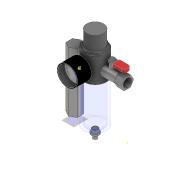
# Autodesk Inventor part: salida_estanque
Saved by Autodesk Inventor 2022 (Build 260153000, 153)
## iProperties
Created: 2022-11-16
Part Number: salida_estanque
Material: Generic
Document SubType Name: Modeling
Designer: ferna
Density: 1 g/cm^3
Appearance: Galvanized
Author: ferna
Autodesk Inventor part; units mm, degrees
ref_plane "YZ Plane" through (0, 0, 0) normal (1, 0, 0) x (0, 1, 0)
ref_plane "XZ Plane" through (0, 0, 0) normal (0, 1, 0) x (-1, 0, 0)
sketch "Sketch1" plane through (0, 0, 0) normal (0, 1, 0) x (-1, 0, 0)
  line L0 (-8, 4.6188) -> (0, 9.2376)
  line L1 (0, 9.2376) -> (8, 4.6188)
  line L2 (8, 4.6188) -> (8, -4.6188)
  line L3 (8, -4.6188) -> (0, -9.2376)
  line L4 (0, -9.2376) -> (-8, -4.6188)
  line L5 (-8, -4.6188) -> (-8, 4.6188)
  point P0 (0, 0)
  point P1 (0, 0)
  dimension "d0" = 8
  constraints: 12 end point, 1 coincident, 13 other
  measures "d0" distance from line of L5 point (0, 0)
extrude "Extrusion1" add sketch "Sketch1" along normal blind 85
sketch "Sketch2" plane through (0, 0, 0) normal (0, -1, 0) x (1, 0, 0)
  circle A0 centre (0, 0) radius 2.5
  dimension "d3" = 5
  constraints: 1 centre point, 1 coincident
  measures "d3" diameter of A0
extrude "Extrusion2" cut sketch "Sketch2" against normal blind 3
sketch "Sketch3" plane through (8, 0, 4.6188) normal (1, 0, 0) x (0, 0, -1)
  circle A0 centre (4.6188, 74.0681) radius 4.2105
  point P0 (4.6188, 0)
  dimension "d22" = 8.4209
  constraints: 1 centre point
  measures "d22" diameter of A0
extrude "Extrusion3" add sketch "Sketch3" along normal blind 5
sketch "Sketch4" plane through (0, 85, 0) normal (0, 1, 0) x (1, 0, 0)
  circle A0 centre (28.9651, 0) radius 15.9651
  point P0 (0, 0)
  constraints: 1 centre point
extrude "Extrusion4" add sketch "Sketch4" along normal blind 10 and the other way blind 25
sketch "Sketch6" plane through (0, 85, 0) normal (0, 1, 0) x (1, 0, 0)
  line L0 (8, 4.5892) -> (13, 4.5892)
  line L1 (13, 4.5892) -> (13, -4.9795)
  line L2 (13, -4.9795) -> (8, -4.9795)
  line L3 (8, -4.9795) -> (8, 4.5892)
  point P0 (0, 0)
  constraints: 8 end point, 2 parallel, 1 horizontal, 1 perpendicular
split body "Split1" sketch "Sketch6" result two bodies curves L2 L3 L0 L1 first body at (-5.0833, 28.3333, 5.7254) (13.7003, 77.7595, -2.4808)
sketch "Sketch7" plane through (28.9651, 95, 0) normal (0, 1, 0) x (1, 0, 0)
  circle A0 centre (0, 0) radius 17.3739
  point P0 (-28.9651, 0)
  constraints: 1 centre point
split body "Split2" sketch "Sketch7" result two bodies bodies 2 curves A0 first body at (44.2299, 71.6667, 2.4808)
sketch "Sketch8" plane through (13, 74.0681, 0) normal (1, 0, 0) x (0, 0, -1)
  circle A0 centre (0, 0) radius 4.2105 projected
  point P0 (0, -74.0681)
extrude "Extrusion5" add sketch "Sketch8" along normal up to surface round surface about axis through (28.9651, 85, 0) along (0, 1, 0) radius 15.9651 far side no bodies 3
sketch "Sketch9" plane through (28.9651, 95, 0) normal (0, 1, 0) x (1, 0, 0)
  circle A0 centre (0, 0) radius 15.9651 projected
  line L0 (0, 15.9651) -> (13.8262, 7.9826)
  line L1 (13.8262, 7.9826) -> (13.8262, -7.9826)
  line L2 (13.8262, -7.9826) -> (0, -15.9651)
  line L3 (0, -15.9651) -> (-13.8262, -7.9826)
  line L4 (-13.8262, -7.9826) -> (-13.8262, 7.9826)
  line L5 (-13.8262, 7.9826) -> (0, 15.9651)
  point P0 (-28.9651, 0)
  constraints: 12 end point, 1 vertical alignment, 14 other
extrude "Extrusion6" add sketch "Sketch9" along normal blind 3 contours L1 L2 L3 L4 L5 L0 bodies 4
sketch "Sketch10" plane through (28.9651, 98, 0) normal (0, 1, 0) x (1, 0, 0)
  circle A0 centre (0, 0) radius 11.9888
  point P0 (-28.9651, 0)
  constraints: 1 centre point
extrude "Extrusion7" add sketch "Sketch10" along normal blind 20 bodies 4
ref_plane "Work Plane1" through (44.9302, 85, 0) normal (1, 0, 0) x (0, 0, -1)
sketch "Sketch11" plane through (44.9302, 85, 0) normal (1, 0, 0) x (0, 0, -1)
  circle A0 centre (0, -10.9319) radius 4.2105 projected
  circle A1 centre (0, -10.9319) radius 7
  point P0 (0, -85)
  dimension "d23" = 14
  constraints: 1 centre point, 1 coincident
  measures "d23" diameter of A1
extrude "Extrusion8" add sketch "Sketch11" along normal blind 30 and the other way blind 10 contours A0 | A1 bodies 5
sketch "Sketch12" plane through (74.9302, 74.0681, 0) normal (1, 0, 0) x (0, 0, -1)
  point P0 (0, -74.0681)
ref_plane "Work Plane2" through (44.9302, 81.0681, 0) normal (0, 1, 0) x (1, 0, 0)
sketch "Sketch13" plane through (44.9302, 81.0681, 0) normal (0, 1, 0) x (1, 0, 0)
  circle A0 centre (8.4764, 0) radius 3.3062
  point P0 (-44.9302, 0)
  constraints: 1 centre point
extrude "Extrusion9" add sketch "Sketch13" along normal blind 12.25 and the other way blind 10 bodies 4
sketch "Sketch14" plane through (74.9302, 74.0681, 0) normal (1, 0, 0) x (0, 0, -1)
  circle A0 centre (0, 0) radius 6
  point P0 (0, -74.0681)
  dimension "d28" = 12
  constraints: 1 centre point
  measures "d28" diameter of A0
extrude "Extrusion10" cut sketch "Sketch14" against normal blind 10 bodies 5
thread "Thread1" size "M12x1.75" class "6H" standard "ANSI Metric M Profile" full length
ref_plane "Work Plane3" through (53.4066, 89.3181, 0) normal (0, 1, 0) x (1, 0, 0)
sketch "Sketch15" plane through (53.4066, 89.3181, 0) normal (0, 1, 0) x (1, 0, 0)
  circle A0 centre (0, 0) radius 3.3062 projected
  circle A1 centre (0, 0) radius 4.3973
  line L0 (0, 4.3973) -> (15.4528, 4.3973)
  line L1 (0, -4.3973) -> (15.4528, -4.3973)
  line L2 (19.9528, 0.1027) -> (19.9528, -0.1027)
  arc A2 (19.9528, -0.1027) -> (15.4528, 4.3973) centre (15.4528, -0.1027) ccw
  arc A3 (15.4528, -4.3973) -> (19.9528, 0.1027) centre (15.4528, 0.1027) ccw
  point P0 (-53.4066, 0)
  point P1 (19.9516, 0)
  dimension "d34" = 4.5
  constraints: 6 end point, 6 point on circle, 5 tangent, 3 centre point, 2 horizontal, 1 coincident, 1 equal radius, 1 perpendicular
  measures "d34" radius of A2
extrude "Extrusion11" add sketch "Sketch15" along normal blind 2 bodies 4
sketch "Sketch16" plane through (0, 0, 0) normal (0, 0, 1) x (1, 0, 0)
  line L0 (13, 60) -> (44.9302, 60) projected
  line L1 (13, 60) -> (13, 0)
  line L2 (13, 0) -> (28.9651, -11.8923)
  line L3 (28.9651, -11.8923) -> (28.9651, -8.5704)
  line L4 (28.9651, -8.5704) -> (16.7121, 0.5567)
  line L5 (16.7121, 0.5567) -> (16.7121, 60)
  line L6 (13, 60) -> (16.7121, 60)
  point P0 (0, 0)
  constraints: 12 end point, 3 parallel, 1 perpendicular, 1 point on line, 1 vertical
revolve "Revolution1" add sketch "Sketch16" angle 360 about axis through (28.9651, -11.8923, 0) along (0, 1, 0) separate body
sketch "Sketch17" plane through (74.9302, 74.0681, 0) normal (1, 0, 0) x (0, 0, -1)
  circle A0 centre (0, 0) radius 4.2105 projected
  line L0 (4.4596, 7.7242) -> (8.9192, 0)
  line L1 (8.9192, 0) -> (4.4596, -7.7242)
  line L2 (4.4596, -7.7242) -> (-4.4596, -7.7242)
  line L3 (-4.4596, -7.7242) -> (-8.9192, 0)
  line L4 (-8.9192, 0) -> (-4.4596, 7.7242)
  line L5 (-4.4596, 7.7242) -> (4.4596, 7.7242)
  circle A1 centre (0, 0) radius 6 projected
  point P0 (0, -74.0681)
  constraints: 12 end point, 1 coincident, 13 other
extrude "Extrusion12" add sketch "Sketch17" against normal blind 10 contours L0 L1 L2 L3 L4 L5 bodies 5
ref_plane "Work Plane4" through (28.9651, 85, 15.9651) normal (0, 0, 1) x (1, 0, 0)
sketch "Sketch19" plane through (28.9651, 85, 15.9651) normal (0, 0, 1) x (1, 0, 0)
  circle A0 centre (0.2293, -5.2602) radius 5.4747
  point P0 (-28.9651, -85)
  dimension "d74" = 10.9494
  constraints: 1 centre point
  measures "d74" diameter of A0
extrude "Extrusion13" add sketch "Sketch19" along normal mid plane 8 separate body
sketch "Sketch20" plane through (29.1944, 79.7398, 19.9651) normal (0, 0, 1) x (1, 0, 0)
  circle A0 centre (0, 0) radius 14.5207
  point P0 (-29.1944, -79.7398)
  dimension "d82" = 29.0415
  constraints: 1 centre point
  measures "d82" diameter of A0
extrude "Extrusion14" add sketch "Sketch20" along normal blind 20 separate body
sketch "Sketch21" plane through (29.1944, 79.7398, 39.9651) normal (0, 0, 1) x (1, 0, 0)
  circle A0 centre (0, 0) radius 13.3396
  point P0 (-29.1944, -79.7398)
  dimension "d83" = 26.6791
  constraints: 1 centre point
  measures "d83" diameter of A0
extrude "Extrusion15" cut sketch "Sketch21" against normal blind 10 bodies 8
sketch "Sketch22" plane through (29.1944, 79.7398, 29.9651) normal (0, 0, 1) x (1, 0, 0)
  line L0 (-16.2249, 17.413) -> (15.7563, 17.413) construction
  line L1 (15.7563, 17.413) -> (15.7563, -16.7823) construction
  line L2 (15.7563, -16.7823) -> (-16.2249, -16.7823) construction
  line L3 (-16.2249, -16.7823) -> (-16.2249, 17.413) construction
  point P0 (-29.1944, -79.7398)
  constraints: 2 other
decal "Decal1"
sketch "Sketch23" plane through (29.1944, 79.7398, 39.9651) normal (0, 0, 1) x (1, 0, 0)
  circle A0 centre (0, 0) radius 13.3396 projected
  point P0 (-29.1944, -79.7398)
extrude "Extrusion16" add sketch "Sketch23" against normal blind 1 separate body
sketch "Sketch24" plane through (28.9651, 60, 0) normal (0, -1, 0) x (1, 0, 0)
  circle A0 centre (0, 0) radius 11.9888 projected
  circle A1 centre (0, 0) radius 4
  point P0 (-28.9651, 0)
  dimension "d61" = 8
  constraints: 1 centre point, 1 coincident
  measures "d61" diameter of A1
extrude "Extrusion17" cut sketch "Sketch24" along normal through all contours A1 bodies 6
ref_plane "Work Plane5" through (0, -9, 0) normal (0, -1, 0) x (1, 0, 0)
sketch "Sketch25" plane through (0, -9, 0) normal (0, -1, 0) x (1, 0, 0)
  circle A0 centre (28.9651, 0) radius 4 projected
  circle A1 centre (28.9651, 0) radius 3.5
  point P0 (0, 0)
  dimension "d65" = 7
  constraints: 1 centre point, 1 coincident
  measures "d65" diameter of A1
extrude "Extrusion18" add sketch "Sketch25" against normal blind 4 bodies 5
sketch "Sketch26" plane through (28.9651, -9, 0) normal (0, -1, 0) x (1, 0, 0)
  circle A0 centre (0, 0) radius 5.5
  point P0 (-28.9651, 0)
  dimension "d68" = 11
  constraints: 1 centre point
  measures "d68" diameter of A0
extrude "Extrusion19" add sketch "Sketch26" along normal blind 2 bodies 5
sketch "Sketch27" plane through (28.9651, -11, 0) normal (0, -1, 0) x (1, 0, 0)
  circle A0 centre (0, 0) radius 3
  point P0 (-28.9651, 0)
  dimension "d71" = 6
  constraints: 1 centre point
  measures "d71" diameter of A0
extrude "Extrusion20" add sketch "Sketch27" along normal blind 6 bodies 5
sketch "Sketch28" plane through (29.1944, 79.7398, 19.9651) normal (0, 0, -1) x (-1, 0, 0)
  circle A0 centre (0, 0) radius 5.4747 projected
  line L0 (7, -7) -> (-7, -7)
  line L1 (-7, -7) -> (-7, 7)
  line L2 (-7, 7) -> (7, 7)
  line L3 (7, 7) -> (7, -7)
  line L4 (7, -7) -> (-7, 7) construction
  line L5 (-7, -7) -> (7, 7) construction
  point P0 (29.1944, -79.7398)
  dimension "d76" = 14
  dimension "d77" = 14
  constraints: 12 end point, 2 midpoint, 2 parallel, 1 horizontal, 1 perpendicular
  measures "d76" distance of L1.end L2.end
  measures "d77" distance of L0.end L1.end
extrude "Extrusion21" add sketch "Sketch28" along normal blind 3 bodies 8
thread "Thread2" size "M11x1.5" class "6g" standard "ANSI Metric M Profile" full length
sketch "Sketch29" plane through (53.4066, 91.3181, 0) normal (0, 1, 0) x (1, 0, 0)
  line L0 (5.6506, 0) -> (5.6506, 5)
  line L1 (15.4528, 4.3973) -> (0, 4.3973) projected
  line L2 (5.6506, 0) -> (10.6506, 0) construction
  line L3 (5.6506, 5) -> (17.6174, 5)
  line L4 (21.5236, 6) -> (11.5236, 6) projected
  line L5 (5.6506, 0) -> (5.6506, -5)
  line L6 (0, -4.3973) -> (15.4528, -4.3973) projected
  line L7 (5.6506, 0) -> (10.6506, 0) construction
  line L8 (5.6506, -5) -> (17.6174, -5)
  arc A0 (17.6174, -5) -> (17.6174, 5) centre (17.6174, 0) ccw
  point P0 (-53.4066, 0)
  dimension "d84" = 5
  dimension "d85" = 90
  dimension "d86" = 5
  dimension "d87" = 90
  constraints: 12 end point, 5 perpendicular, 2 horizontal, 2 point on circle, 2 tangent, 1 centre point, 1 parallel
  measures "d84" distance of L0.start L0.end
  measures "d85" angle of L2 L0
  measures "d86" distance of L0.start L5.end
  measures "d87" angle of L5 L7
extrude "Extrusion22" add sketch "Sketch29" along normal blind 1 and the other way blind 3 separate body
body "Solid6"
body "Solid7"
body "Solid8"
body "Solid9"
body "Solid10"
body "Solid3"
body "Solid4"
body "Solid5"
